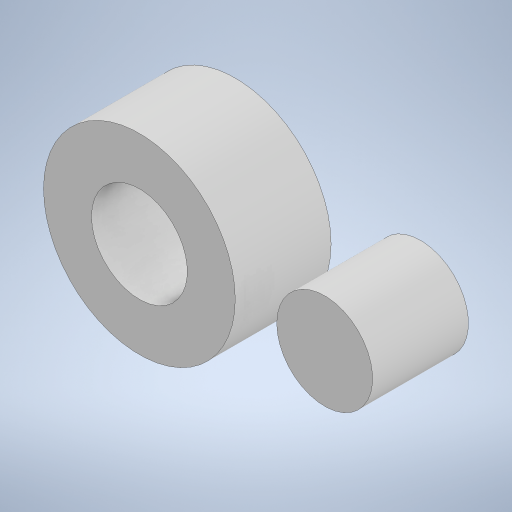
# Autodesk Inventor part: Part1
Saved by Autodesk Inventor 2024 (Build 280153000, 153)
## iProperties
Created: 2023-12-24
Part Number: Part1
Material: Generic
Document SubType Name: Modeling
Designer: jebes windows
Density: 1 g/cm^3
Appearance: Default
Author: jebes windows
Autodesk Inventor part; units mm, degrees
ref_plane "YZ Plane" through (0, 0, 0) normal (1, 0, 0) x (0, 1, 0)
ref_plane "XZ Plane" through (0, 0, 0) normal (0, 1, 0) x (-1, 0, 0)
ref_plane "XY Plane" through (0, 0, 0) normal (0, 0, 1) x (1, 0, 0)
sketch "Sketch1" plane through (0, 0, 0) normal (0, 1, 0) x (-1, 0, 0)
  circle A0 centre (0, 0) radius 2.5
  circle A1 centre (9.6653, 0) radius 2.5
  circle A2 centre (9.6653, 0) radius 5
  dimension "d0" = 5
  dimension "d1" = 5
  dimension "d2" = 10
  dimension "d3" = 9.6653
  constraints: 3 centre point, 2 coincident, 1 horizontal alignment
  measures "d0" diameter of A0
  measures "d1" diameter of A1
  measures "d2" diameter of A2
  measures "d3" distance of point (0, 0) A1.centre
extrude "Extrusion1" add sketch "Sketch1" along normal blind 5
body "Solid1"
